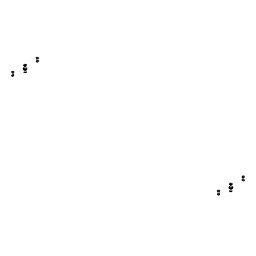
Shelf support D5 L16 with additional holes (Autodesk Fusion 360 design; units mm, degrees)
description: Shelf support D5 L16
Autodesk Fusion 360 part; units mm, degrees
sketch "Contact Area" plane through (0, 0, 0) normal (0, 0, 1) x (1, 0, 0)
  line L0 (300, -9) -> (-300, -9)
  line L1 (-300, -9) -> (-300, 9)
  line L2 (-300, 9) -> (300, 9)
  line L3 (300, 9) -> (300, -9)
  line L4 (300, -9) -> (-300, 9) construction
  line L5 (-300, -9) -> (300, 9) construction
  dimension "d3" = 600
  dimension "d4" = 18
  constraint horizontal L0
  constraint perpendicular L0 L1
  constraint parallel L0 L2
  constraint parallel L1 L3
  constraint coincident L4 origin
  constraint coincident L5 origin
  measures "d3" distance of L0.start L0.end
  measures "d4" distance of L0.end L1.end
sketch "Sketch2" plane through (0, 0, 0) normal (0, 0, 1) x (1, 0, 0)
  circle A0 centre (-268, 11.5) radius 2.5
  line L0 (300, -9) -> (-300, -9)
  line L1 (-300, -9) -> (-300, 9)
  circle A1 centre (268, 11.5) radius 2.5
  line L2 (300, 9) -> (300, -9)
  line L3 (-300, 9) -> (300, 9)
  dimension "d5" = 5
  dimension "d7" = 32
  dimension "d8" = 32
  constraint equal A0 A1
  constraint tangent A0 L3
  constraint tangent A1 L3
  measures "d5" diameter of A0
  measures "d7" distance of A0.centre L1
  measures "d8" distance of A1.centre L2
extrude "Extrude1" add sketch "Sketch2" along normal blind 7.5 contours A0 makes body 1
chamfer "Chamfer1" distance 0.5 angle 45 1 edges at (-270.3308, 10.596, 7.5) on bodies 1
sketch "Sketch3" plane through (0, 0, 0) normal (0, 0, -1) x (-1, 0, 0)
  circle A0 centre (268, 11.5) radius 2.5
  circle A1 centre (268, 11.5) radius 3.5
  dimension "d12" = 7
  constraint concentric A0 A1
  measures "d12" diameter of A1
extrude "Extrude2" add sketch "Sketch3" along normal blind 1 contours A0 | A1 bodies 1
sketch "Sketch4" plane through (0, 0, -1) normal (0, 0, -1) x (-1, 0, 0)
  circle A0 centre (268, 11.5) radius 3.5
  circle A1 centre (268, 11.5) radius 2.5
  dimension "d15" = 5
  constraint concentric A0 A1
  measures "d15" diameter of A1
extrude "Extrude3" add sketch "Sketch4" along normal blind 7.5 contours A1 bodies 1
chamfer "Chamfer2" distance 0.5 angle 45 1 edges at (-265.6692, 10.596, -8.5) on bodies 1
copy_body "Body->Comp1" bodies 1 removing the originals makes body 2 in component "Shelf support D5 L16"
sketch "Sketch1" plane through (0, 0, -1) normal (0, 0, -1) x (1, 0, 0) in component "Shelf support D5 L16"
  circle A0 centre (-268, -11.5) radius 2.5
  circle A1 centre (-268, -11.5) radius 3.5
  circle A2 centre (-268, -11.5) radius 2.5
  dimension "d27" = 5
  constraint concentric A0 A2
  measures "d27" diameter of A2
extrude "Extrude1'" add sketch "Sketch1" along normal blind 8 separate body contours A0 A2 makes body 3 in component "Shelf support D5 L16"
copy_body "Body->Comp1'" bodies 3 removing the originals makes body 4 in component "Hole"
pattern_linear "00000000-0000-0000-0000-000000000000" [suppressed] in component "Shelf support D5 L16"
component "Shelf support D5 L16" placed x (1, 0, 0) y (0, -1, 0) z (0, 0, -1) at (0, 23, -1)
component "Shelf support D5 L16" placed x (1, 0, 0) y (0, -1, 0) z (0, 0, -1) at (536, 23, -1)
component "Hole" placed x (1, 0, 0) y (0, 1, 0) z (0, 0, 1) at (0, 0, 0) in component "Shelf support D5 L16"
component "Hole" placed x (1, 0, 0) y (0, 1, 0) z (0, 0, 1) at (0, 32, 0) in component "Shelf support D5 L16"
component "Hole" placed x (1, 0, 0) y (0, 1, 0) z (0, 0, 1) at (0, -32, 0) in component "Shelf support D5 L16"
component "Hole" placed x (1, 0, 0) y (0, 1, 0) z (0, 0, 1) at (0, 32, 0) in component "Shelf support D5 L16"
component "Hole" placed x (1, 0, 0) y (0, 1, 0) z (0, 0, 1) at (0, -32, 0) in component "Shelf support D5 L16"
equation "ContactAreaLength = 600 mm" comment "Contact Area Length"
equation "ContactAreaWidth = 18 mm" comment "Pillar Board Thickness"
equation "d3 = ContactAreaLength"
equation "d4 = ContactAreaWidth"
equation "DistFromEdge = 32 mm" comment "Distance From Edge(s)"
equation "d7 = DistFromEdge"
equation "d8 = DistFromEdge"
equation "Holes_qty = 3"
equation "d35 = Holes_qty"
equation "d37 = Dist_between_holes"
equation "d39 = Holes_qty"
equation "Dist_between_holes = 32 mm"
named bodies: "Shelf support D5 L16", "Hole"
